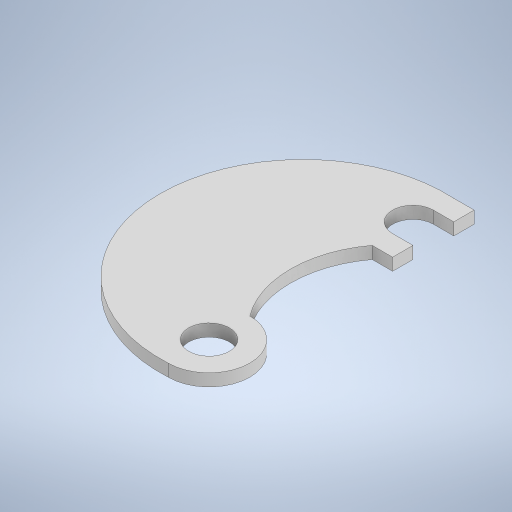
# Autodesk Inventor part: key
Saved by Autodesk Inventor 2023 (Build 270158030, 158C)
## iProperties
Created: 2023-03-06
Part Number: key
Material: Generic
Document SubType Name: Modeling
Designer: fatih
Density: 1 g/cm^3
Appearance: Default
Author: fatih
Autodesk Inventor part; units mm, degrees
ref_plane "YZ Plane" through (0, 0, 0) normal (1, 0, 0) x (0, 1, 0)
ref_plane "XZ Plane" through (0, 0, 0) normal (0, 1, 0) x (-1, 0, 0)
ref_plane "XY Plane" through (0, 0, 0) normal (0, 0, 1) x (1, 0, 0)
sketch "Sketch1" plane through (0, 0, 0) normal (0, 1, 0) x (-1, 0, 0)
  circle A0 centre (0, 0) radius 5
  circle A1 centre (0, 0) radius 10
  arc A2 (0, -55) -> (0, -45) centre (0, -50) ccw
  line L0 (0, -55) -> (-5, -55)
  line L1 (-5, -55) -> (-5, -60)
  line L2 (-5, -60) -> (0, -60)
  line L3 (0, -60) -> (0, -55)
  line L4 (0, -45) -> (-5, -45)
  line L5 (-5, -45) -> (-5, -40)
  line L6 (-5, -40) -> (0, -40)
  line L7 (0, -40) -> (0, -45)
  arc A3 (0, -40) -> (0, -10) centre (-19.9855, -25) ccw
  arc A4 (0, -60) -> (0, 10) centre (1.9294, -25) ccw
  dimension "d9" = 10
  dimension "d10" = 20
  dimension "d12" = 5
  dimension "d13" = 5
  dimension "d14" = 5
  dimension "d15" = 5
  constraints: 16 end point, 8 point on circle, 5 centre point, 4 parallel, 2 horizontal, 2 perpendicular, 1 coincident
  measures "d9" diameter of A0
  measures "d10" diameter of A1
  measures "d12" distance of L2.end L1.end
  measures "d13" distance of L1.end L0.end
  measures "d14" distance of L5.end L6.end
  measures "d15" distance of L4.end L5.end
extrude "Extrusion2" add sketch "Sketch1" along normal blind 3
body "Solid2"
